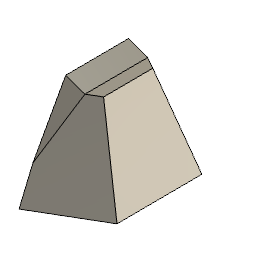
cncmold (Autodesk Fusion 360 design; units mm, degrees)
part number: 2025-10-25-13-18-41-276
Autodesk Fusion 360 part; units mm, degrees
sketch "Sketch1" plane through (0, 0, 0) normal (0, 0, 1) x (1, 0, 0)
  line L0 (43.7079, 24.2821) -> (0.825, 49.9932)
  line L1 (-0.825, -49.9932) -> (42.8829, -25.711)
  line L2 (42.8829, -25.711) -> (43.7079, 24.2821)
  line L3 (0.825, 49.9932) -> (0.825, -49.0766)
  dimension "d1" = 50
  constraint coincident L1 L3.end
  constraint vertical L3
  measures "d1" distance of L0.start origin
sketch "Sketch2" plane through (0, 0, 0) normal (0, 0, 1) x (1, 0, 0)
  line L0 (143.1555, 105.2509) -> (99.7098, 129.9992)
  line L1 (100.2902, 30.0008) -> (143.4456, 55.2517)
  line L2 (143.4456, 55.2517) -> (143.1555, 105.2509)
  line L3 (99.7098, 129.9992) -> (100.2902, 30.0008)
  point P0 (100, 80)
  dimension "d8" = 50
  measures "d8" distance of L0.start P0
extrude "Extrude2" add sketch "Sketch2" along normal blind 50 draft -20
extrude "Extrude3" add 1 faces at (106.1018, 73.8756, 16.6667) along direction (-0.939677, -0.005453, 0.34202) blind 20
extrude "Extrude4" add 1 faces at (87.5677, 63.2609, 4.5603) along direction (-0.342014, -0.001985, -0.939693) blind 10
sketch "Sketch3" plane through (-0.7511, 129.4161, 0) normal (-0.005803, 0.999983, 0) x (-0.999983, -0.005803, 0)
  line L0 (-81.6687, 6.8404) -> (-100.4626, 0)
  line L1 (-100.4626, 0) -> (-97.0424, -9.3969)
  line L2 (-97.0424, -9.3969) -> (-78.2485, -2.5565)
  line L3 (-78.2485, -2.5565) -> (-81.6687, 6.8404)
  line L4 (-100.4626, 0) -> (-74.4233, 0)
  line L5 (-74.4233, 0) -> (-74.4233, -10.8418)
  line L6 (-74.4233, -10.8418) -> (-100.4626, -10.8418)
  line L7 (-100.4626, -10.8418) -> (-100.4626, 0)
  line L8 (-100.4626, 0) -> (-74.4413, 0)
  line L9 (-74.4413, 0) -> (-74.4413, 61.5584)
  line L10 (-74.4413, 61.5584) -> (-100.4626, 61.5584)
  line L11 (-100.4626, 61.5584) -> (-100.4626, 0)
  constraint horizontal L4
  constraint vertical L5
  constraint horizontal L6
  constraint vertical L7
  constraint coincident L0.end L1.start
  constraint horizontal L8
  constraint vertical L9
  constraint horizontal L10
  constraint vertical L11
extrude "Extrude5" cut sketch "Sketch3" against normal blind 100
extrude "Extrude8" cut 1 faces at (100.0357, 73.8404, 18.8746) along direction (0.999983, 0.005803, 0) blind 7
